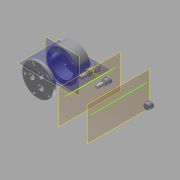
# Autodesk Inventor part: Filtration_tube
Saved by Autodesk Inventor 2012 (Build 160160000, 160)
## iProperties
Created: 2012-10-07
Part Number: Filtration_tube
Material: Default
Document SubType Name: Modeling
Designer: Dazed
Density: 1 g/cm^3
Author: Dazed
Autodesk Inventor part; units mm, degrees
ref_plane "YZ Plane" through (0, 0, 0) normal (1, 0, 0) x (0, 1, 0)
ref_plane "XZ Plane" through (0, 0, 0) normal (0, 1, 0) x (-1, 0, 0)
ref_plane "XY Plane" through (0, 0, 0) normal (0, 0, 1) x (1, 0, 0)
sketch "Sketch1" plane through (0, 0, 0) normal (0, 0, 1) x (1, 0, 0)
  circle A0 centre (0, 0) radius 38.1
  dimension "d0" = 76.2
  constraints: 1 centre point
  measures "d0" diameter of A0
extrude "Extrusion1" add sketch "Sketch1" along normal blind 7.62
sketch "Sketch2" plane through (0, 0, 7.62) normal (0, 0, 1) x (1, 0, 0)
  circle A0 centre (0, 0) radius 38.1 projected
  line L0 (-28.2512, -2.02) -> (-31.75, -4.0401)
  line L1 (-31.75, -4.0401) -> (-35.2488, -2.02)
  line L2 (-35.2488, -2.02) -> (-35.2488, 2.02)
  line L3 (-35.2488, 2.02) -> (-31.75, 4.0401)
  line L4 (-31.75, 4.0401) -> (-28.2512, 2.02)
  line L5 (-28.2512, 2.02) -> (-28.2512, -2.02)
  line L6 (-6.8089, -27.4927) -> (-5.969, -31.4445)
  line L7 (-5.969, -31.4445) -> (-8.9713, -34.1478)
  line L8 (-8.9713, -34.1478) -> (-12.8136, -32.8994)
  line L9 (-12.8136, -32.8994) -> (-13.6536, -28.9476)
  line L10 (-13.6536, -28.9476) -> (-10.6513, -26.2443)
  line L11 (-10.6513, -26.2443) -> (-6.8089, -27.4927)
  line L12 (24.043, -14.9714) -> (28.061, -15.3937)
  line L13 (28.061, -15.3937) -> (29.7042, -19.0845)
  line L14 (29.7042, -19.0845) -> (27.3295, -22.353)
  line L15 (27.3295, -22.353) -> (23.3116, -21.9307)
  line L16 (23.3116, -21.9307) -> (21.6684, -18.2399)
  line L17 (21.6684, -18.2399) -> (24.043, -14.9714)
  line L18 (21.6684, 18.2399) -> (23.3116, 21.9307)
  line L19 (23.3116, 21.9307) -> (27.3295, 22.353)
  line L20 (27.3295, 22.353) -> (29.7042, 19.0845)
  line L21 (29.7042, 19.0845) -> (28.061, 15.3937)
  line L22 (28.061, 15.3937) -> (24.043, 14.9714)
  line L23 (24.043, 14.9714) -> (21.6684, 18.2399)
  line L24 (-10.6513, 26.2443) -> (-13.6536, 28.9476)
  line L25 (-13.6536, 28.9476) -> (-12.8136, 32.8994)
  line L26 (-12.8136, 32.8994) -> (-8.9713, 34.1478)
  line L27 (-8.9713, 34.1478) -> (-5.969, 31.4445)
  line L28 (-5.969, 31.4445) -> (-6.8089, 27.4927)
  line L29 (-6.8089, 27.4927) -> (-10.6513, 26.2443)
  point P0 (-31.75, 0)
  point P1 (-9.8113, -30.196)
  point P2 (25.6863, -18.6622)
  point P3 (25.6863, 18.6622)
  point P4 (-9.8113, 30.196)
  dimension "d8" = 360
  constraints: 60 end point, 79 other
extrude "Extrusion2" cut sketch "Sketch2" against normal blind 2.8829 contours L0 L1 L2 L3 L4 L5 | L6 L7 L8 L9 L10 L11 | L12 L13 L14 L15 L16 L17 | L18 L19 L20 L21 L22 L23 | L24 L25 L26 L27 L28 L29
sketch "Sketch3" plane through (0, 0, 7.62) normal (0, 0, 1) x (1, 0, 0)
  circle A0 centre (0, 0) radius 38.1 projected
  circle A1 centre (-31.75, 0) radius 2.0066
  circle A2 centre (-9.8113, -30.196) radius 2.0066
  circle A3 centre (25.6863, -18.6622) radius 2.0066
  circle A4 centre (25.6863, 18.6622) radius 2.0066
  circle A5 centre (-9.8113, 30.196) radius 2.0066
  dimension "d12" = 31.75
  dimension "d13" = 4.0132
  dimension "d16" = 360
  constraints: 5 centre point, 11 other
  measures "d12" distance of A0.centre A1.centre
  measures "d13" diameter of A1
extrude "Extrusion3" cut sketch "Sketch3" against normal blind 10.16 contours A1 | A2 | A3 | A4 | A5
ref_plane "Work Plane1" through (0, 0, -52.3875) normal (0, 0, -1) x (-1, 0, 0)
sketch "Sketch4" plane through (0, 0, -52.3875) normal (0, 0, -1) x (-1, 0, 0)
  circle A0 centre (0, 0) radius 38.1 projected
  circle A1 centre (-25.6863, 18.6622) radius 2.0066 projected
  circle A2 centre (9.8113, 30.196) radius 2.0066 projected
  circle A3 centre (31.75, 0) radius 2.0066 projected
  circle A4 centre (9.8113, -30.196) radius 2.0066 projected
  circle A5 centre (-25.6863, -18.6622) radius 2.0066 projected
  circle A6 centre (0, 0) radius 26.9875
  dimension "d21" = 53.975
  constraints: 1 centre point
  measures "d21" diameter of A6
extrude "Extrusion4" add sketch "Sketch4" along normal blind 25.4
sketch "Sketch5" plane through (0, 0, -77.7875) normal (0, 0, -1) x (-1, 0, 0)
  circle A0 centre (-25.6863, -18.6622) radius 2.0066 projected
  circle A1 centre (9.8113, -30.196) radius 2.0066 projected
  circle A2 centre (31.75, 0) radius 2.0066 projected
  circle A3 centre (9.8113, 30.196) radius 2.0066 projected
  circle A4 centre (-25.6863, 18.6622) radius 2.0066 projected
  circle A5 centre (0, 0) radius 38.1 projected
extrude "Extrusion5" add sketch "Sketch5" along normal blind 6.35
sketch "Sketch6" plane through (0, 0, 7.62) normal (0, 0, 1) x (1, 0, 0)
  circle A0 centre (0, 0) radius 38.1 projected
  circle A1 centre (-14.8844, 0) radius 6.731
  circle A2 centre (7.4422, -12.8903) radius 6.731
  circle A3 centre (7.4422, 12.8903) radius 6.731
  dimension "d26" = 13.462
  dimension "d27" = 14.8844
  dimension "d30" = 360
  constraints: 3 centre point, 7 other
  measures "d26" diameter of A1
  measures "d27" distance of A0.centre A1.centre
extrude "Extrusion6" cut sketch "Sketch6" against normal blind 10.16 contours A1 | A2 | A3
sketch "Sketch7" plane through (0, 0, -52.3875) normal (0, 0, -1) x (-1, 0, 0)
  circle A0 centre (-62.882, 16.0283) radius 6.731
  circle A1 centre (-7.4422, 12.8903) radius 6.731 projected
  circle A2 centre (-62.882, 16.0283) radius 2.921
  point P0 (0, 0)
  dimension "d34" = 13.462
  dimension "d35" = 13.462
  dimension "d36" = 5.842
  constraints: 2 centre point
  measures "d34" diameter of A0
  measures "d35" diameter of A1
  measures "d36" diameter of A2
extrude "Extrusion7" add sketch "Sketch7" along normal blind 7.62 contours A0
sketch "Sketch8" plane through (62.882, 16.0283, -60.0075) normal (0, 0, -1) x (-1, 0, 0)
  circle A0 centre (0, 0) radius 2.921 projected
  circle A1 centre (0, 0) radius 6.731 projected
  line L0 (-15.8316, 0) -> (11.9547, 0)
  point P0 (62.882, -16.0283)
  constraints: 2 end point
ref_plane "Work Plane2" through (78.7135, 16.0283, -60.0075) normal (0, -1, 0) x (-1, 0, 0)
sketch "Sketch9" plane through (78.7135, 16.0283, -60.0075) normal (0, -1, 0) x (-1, 0, 0)
  arc A0 (15.8316, 20.7645) -> (7.7671, 12.7) centre (15.8316, 12.7) ccw
  line L0 (7.7671, 12.7) -> (7.7671, 0)
  line L1 (12.9106, 3.81) -> (12.9106, -20.4154)
  line L2 (9.1006, 3.81) -> (12.9106, 3.81)
  line L3 (10.8663, 0) -> (12.9106, 0)
  line L4 (18.7526, 0) -> (21.4872, 0)
  line L5 (7.7671, 0) -> (12.9106, 0)
  line L6 (18.7526, 0) -> (23.8961, 0)
  line L7 (9.1006, 3.81) -> (9.1006, 12.7)
  arc A1 (15.8316, 19.431) -> (9.1006, 12.7) centre (15.8316, 12.7) ccw
  line L8 (15.8316, 19.431) -> (15.8316, 20.7645)
  line L9 (7.7671, 0) -> (12.9106, 0)
  point P0 (78.7135, -60.0075)
  constraints: 20 end point, 4 point on circle, 2 centre point, 1 point on line, 1 tangent
revolve "Revolution1" add sketch "Sketch9" angle 360 about axis through (62.882, 16.0283, -79.4385) along (0, 0, -1)
sketch "Sketch10" plane through (62.882, 16.0283, -60.0075) normal (0, 0, 1) x (1, 0, 0)
  line L0 (-3.0668, 0.8218) -> (-8.8573, 2.3733)
  line L1 (-2.9226, 1.2406) -> (-8.4408, 3.5829)
  line L2 (0, 0) -> (-9.1697, 0)
  line L3 (-2.5019, 1.9547) -> (-7.2259, 5.6455)
  line L4 (-2.2055, 2.2839) -> (-6.3698, 6.5962)
  line L5 (0, 3.175) -> (0, 13.2072)
  line L6 (3.0668, 0.8218) -> (8.8573, 2.3733)
  line L7 (2.9226, 1.2406) -> (8.4408, 3.5829)
  line L8 (2.5019, 1.9547) -> (7.2259, 5.6455)
  line L9 (2.2055, 2.2839) -> (6.3698, 6.5962)
  line L10 (-1.5393, 2.7769) -> (-4.4456, 8.02)
  line L11 (-1.1378, 2.9641) -> (-3.2861, 8.5607)
  line L12 (-0.7142, 3.0936) -> (-2.0627, 8.9347)
  line L13 (-0.2767, 3.1629) -> (-0.7992, 9.1348)
  line L14 (1.5393, 2.7769) -> (4.4456, 8.02)
  line L15 (1.1378, 2.9641) -> (3.2861, 8.5607)
  line L16 (0.7142, 3.0936) -> (2.0627, 8.9347)
  line L17 (0.2767, 3.1629) -> (0.7992, 9.1348)
  line L18 (-3.0668, -0.8218) -> (-8.8573, -2.3733)
  line L19 (-2.9226, -1.2406) -> (-8.4408, -3.5829)
  line L20 (-2.5019, -1.9547) -> (-7.2259, -5.6455)
  line L21 (-2.2055, -2.2839) -> (-6.3698, -6.5962)
  line L22 (3.0668, -0.8218) -> (8.8573, -2.3733)
  line L23 (2.9226, -1.2406) -> (8.4408, -3.5829)
  line L24 (2.5019, -1.9547) -> (7.2259, -5.6455)
  line L25 (2.2055, -2.2839) -> (6.3698, -6.5962)
  line L26 (-1.5393, -2.7769) -> (-4.4456, -8.02)
  line L27 (-1.1378, -2.9641) -> (-3.2861, -8.5607)
  line L28 (-0.7142, -3.0936) -> (-2.0627, -8.9347)
  line L29 (-0.2767, -3.1629) -> (-0.7992, -9.1348)
  line L30 (1.5393, -2.7769) -> (4.4456, -8.02)
  line L31 (1.1378, -2.9641) -> (3.2861, -8.5607)
  line L32 (0.7142, -3.0936) -> (2.0627, -8.9347)
  line L33 (0.2767, -3.1629) -> (0.7992, -9.1348)
  circle A0 centre (0, 0) radius 3.175
  arc A1 (-8.8573, -2.3733) -> (-8.4408, -3.5829) centre (0, 0) ccw
  arc A2 (-7.2259, -5.6455) -> (-6.3698, -6.5962) centre (0, 0) ccw
  arc A3 (-4.4456, -8.02) -> (-3.2861, -8.5607) centre (0, 0) ccw
  arc A4 (-2.0627, -8.9347) -> (-0.7992, -9.1348) centre (0, 0) ccw
  arc A5 (0.7992, -9.1348) -> (2.0627, -8.9347) centre (0, 0) ccw
  arc A6 (3.2861, -8.5607) -> (4.4456, -8.02) centre (0, 0) ccw
  arc A7 (6.3698, -6.5962) -> (7.2259, -5.6455) centre (0, 0) ccw
  arc A8 (8.4408, -3.5829) -> (8.8573, -2.3733) centre (0, 0) ccw
  arc A9 (8.8573, 2.3733) -> (8.4408, 3.5829) centre (0, 0) ccw
  arc A10 (7.2259, 5.6455) -> (6.3698, 6.5962) centre (0, 0) ccw
  arc A11 (4.4456, 8.02) -> (3.2861, 8.5607) centre (0, 0) ccw
  arc A12 (2.0627, 8.9347) -> (0.7992, 9.1348) centre (0, 0) ccw
  arc A13 (-0.7992, 9.1348) -> (-2.0627, 8.9347) centre (0, 0) ccw
  arc A14 (-3.2861, 8.5607) -> (-4.4456, 8.02) centre (0, 0) ccw
  arc A15 (-6.3698, 6.5962) -> (-7.2259, 5.6455) centre (0, 0) ccw
  arc A16 (-8.4408, 3.5829) -> (-8.8573, 2.3733) centre (0, 0) ccw
  point P0 (-62.882, -16.0283)
  point P1 (-10.688, 2.8638)
  point P2 (-10.6991, 4.5415)
  point P3 (-8.6178, 6.733)
  point P4 (-7.072, 7.3233)
  point P5 (10.688, 2.8638)
  point P6 (10.6991, 4.5415)
  point P7 (8.6178, 6.733)
  point P8 (7.072, 7.3233)
  point P9 (-5.2155, 9.409)
  point P10 (-4.1427, 10.792)
  point P11 (-3.1438, 13.6174)
  point P12 (-1.2316, 14.0771)
  point P13 (5.2155, 9.409)
  point P14 (4.1427, 10.792)
  point P15 (3.1438, 13.6174)
  point P16 (1.2316, 14.0771)
  point P17 (-10.688, -2.8638)
  point P18 (-10.6991, -4.5415)
  point P19 (-8.6178, -6.733)
  point P20 (-7.072, -7.3233)
  point P21 (10.688, -2.8638)
  point P22 (10.6991, -4.5415)
  point P23 (8.6178, -6.733)
  point P24 (7.072, -7.3233)
  point P25 (-5.2155, -9.409)
  point P26 (-4.1427, -10.792)
  point P27 (-3.1438, -13.6174)
  point P28 (-1.2316, -14.0771)
  point P29 (5.2155, -9.409)
  point P30 (4.1427, -10.792)
  point P31 (3.1438, -13.6174)
  point P32 (1.2316, -14.0771)
  dimension "d58" = 6.35
  dimension "d50" = 15
  dimension "d51" = 8
  dimension "d52" = 15
  dimension "d53" = 8
  dimension "d54" = 15
  dimension "d55" = 8
  dimension "d56" = 8
  dimension "d57" = 8
  constraints: 68 end point, 32 point on circle, 24 symmetric about line, 16 centre point, 1 horizontal, 35 other
  measures "d50" angle of L2 L0
  measures "d51" angle of L1 L0
  measures "d52" angle of L3 L1
  measures "d53" angle of L4 L3
  measures "d54" angle of L10 L4
  measures "d55" angle of L11 L10
  measures "d56" angle of L12 L11
  measures "d57" angle of L13 L12
extrude "Extrusion8" cut sketch "Sketch10" against normal blind 25.4 contours L0 A16 L1 A0 | L3 A15 L4 A0 | A0 L19 A1 L18 | L10 A14 L11 A0 | A0 L21 A2 L20 | L12 A13 L13 A0 | A0 L27 A3 L26 | A0 L29 A4 L28 | L17 A12 L16 A0 | A0 L32 A5 L33 | L15 A11 L14 A0 | A0 L30 A6 L31 | L9 A10 L8 A0 | A0 L24 A7 L25 | L7 A9 L6 A0 | A0 L22 A8 L23
sketch "Sketch11" plane through (62.882, 16.0283, -63.8175) normal (0, 0, -1) x (-1, 0, 0)
  circle A0 centre (0, 0) radius 2.921 projected
  circle A1 centre (0, 0) radius 8.0645
  point P0 (62.882, -16.0283)
  dimension "d61" = 16.129
  constraints: 1 centre point
  measures "d61" diameter of A1
extrude "Extrusion9" add sketch "Sketch11" against normal blind 3.81
sketch "Sketch13" plane through (78.7135, 16.0283, -60.0075) normal (0, -1, 0) x (-1, 0, 0)
  line L0 (18.7526, -7.62) -> (12.9106, -7.62) projected
  line L1 (15.8316, -29.7183) -> (15.8316, 1.013)
  line L2 (12.9106, -26.3367) -> (12.9106, -7.62)
  line L3 (12.0216, -26.3367) -> (11.2596, -24.8419)
  line L4 (11.2596, -24.8419) -> (11.2596, -22.6148)
  line L5 (11.2596, -22.6148) -> (12.0216, -23.119)
  line L6 (12.0216, -26.3367) -> (12.9106, -26.3367)
  line L7 (12.0216, -21.1629) -> (11.2596, -19.668)
  line L8 (11.2596, -19.668) -> (11.2596, -17.4409)
  line L9 (11.2596, -17.4409) -> (12.0216, -17.9452)
  line L10 (12.0216, -16.501) -> (11.2596, -15.0062)
  line L11 (11.2596, -15.0062) -> (11.2596, -12.779)
  line L12 (11.2596, -12.779) -> (12.0216, -13.2833)
  line L13 (11.2596, -10.7157) -> (11.2596, -7.2324)
  line L14 (11.2596, -7.62) -> (12.9106, -7.62)
  line L15 (11.2596, -10.7157) -> (12.0851, -10.7157)
  line L16 (12.0216, -10.7157) -> (12.0216, -13.2833)
  line L17 (12.0216, -16.501) -> (12.0216, -17.9452)
  line L18 (12.0216, -21.1629) -> (12.0216, -23.119)
  point P0 (78.7135, -60.0075)
  dimension "d65" = 4.572
  constraints: 36 end point, 3 point on line, 1 vertical
  measures "d65" distance between parallel lines of L4 L1
revolve "Revolution2" add sketch "Sketch13" angle 360 about axis through (62.882, 16.0283, -30.2892) along (0, 0, -1)
sketch "Sketch14" plane through (78.7135, 16.0283, -60.0075) normal (0, -1, 0) x (-1, 0, 0)
  line L0 (-4.3063, 38.8955) -> (-4.3063, -86.0346)
  line L1 (-75.6718, 44.7873) -> (-75.6718, -93.7628)
  point P0 (78.7135, -60.0075)
  constraints: 4 end point
ref_plane "Work Plane3" through (83.0198, 16.0283, -98.903) normal (1, 0, 0) x (0, 0, 1)
ref_plane "Work Plane4" through (154.3853, 16.0283, -104.7948) normal (1, 0, 0) x (0, 0, 1)
mirror "Mirror1" about plane through (83.0198, 16.0283, -98.903) normal (1, 0, 0) of "Extrusion8", "Revolution1", "Extrusion7", "Revolution2", "Extrusion9"
sketch "Sketch15" plane through (103.1577, 16.0283, -63.8175) normal (0, 0, -1) x (-1, 0, 0)
  line L0 (9.9671, 17.9811) -> (-10.9543, 17.9811)
  line L1 (-10.9543, 17.9811) -> (-10.9543, -12.2992)
  line L2 (-10.9543, -12.2992) -> (9.9671, -12.2992)
  line L3 (9.9671, -12.2992) -> (9.9671, 17.9811)
  point P0 (103.1577, -16.0283)
  constraints: 8 end point, 2 parallel, 1 horizontal, 1 perpendicular
extrude "Extrusion10" cut sketch "Sketch15" along normal blind 25.4
mirror "Mirror2" about plane through (154.3853, 16.0283, -104.7948) normal (1, 0, 0) of "Extrusion10", "Extrusion8", "Revolution1", "Extrusion7", "Revolution2", "Extrusion9", "Mirror1"
sketch "Sketch16" plane through (205.613, 16.0283, -52.3875) normal (0, 0, 1) x (1, 0, 0)
  line L0 (-18.5986, 17.2513) -> (23.2617, 17.2513)
  line L1 (23.2617, 17.2513) -> (23.2617, -16.0283)
  line L2 (23.2617, -16.0283) -> (-18.5986, -16.0283)
  line L3 (-18.5986, -16.0283) -> (-18.5986, 17.2513)
  point P0 (-205.613, -16.0283)
  constraints: 8 end point, 2 parallel, 1 horizontal, 1 perpendicular
extrude "Extrusion11" cut sketch "Sketch16" along normal blind 25.4
sketch "Sketch17" plane through (205.613, 16.0283, -52.3875) normal (0, 0, 1) x (1, 0, 0)
  circle A0 centre (0, 0) radius 2.921 projected
  point P0 (-205.613, -16.0283)
extrude "Extrusion12" add sketch "Sketch17" against normal blind 11.43
sketch "Sketch18" plane through (205.613, 16.0283, -63.8175) normal (0, 0, -1) x (-1, 0, 0)
  line L0 (-26.6027, 21.4545) -> (-61.3931, 21.4545)
  line L1 (-61.3931, 21.4545) -> (-61.3931, -31.7158)
  line L2 (-61.3931, -31.7158) -> (-26.6027, -31.7158)
  line L3 (-26.6027, -31.7158) -> (-26.6027, 21.4545)
  point P0 (205.613, -16.0283)
  constraints: 8 end point, 2 parallel, 1 horizontal, 1 perpendicular
extrude "Extrusion13" cut sketch "Sketch18" along normal mid plane 76.2
equation "\"d34\" = d35"
body "Solid1"
